Autodesk Inventor part; units mm, degrees
(part 2 of 2)
sketch "Sketch23" plane through (-20, 0, 0) normal (-1, 0, 0) x (0, 0, 1)
  circle A0 centre (8.0719, -81.9132) radius 5.7664 projected
  circle A1 centre (83.0719, -81.9132) radius 3.9821 projected
  circle A2 centre (2.2876, 58.0868) radius 3 projected
  circle A3 centre (83.0715, 100.0868) radius 3 projected
  circle A4 centre (83.0715, 260.0868) radius 3 projected
  circle A5 centre (8.0719, 243.0868) radius 2.5 projected
  circle A6 centre (37.6815, 343.0868) radius 3 projected
  circle A7 centre (83.0719, 348.0868) radius 6.7103 projected
  point P0 (0, 0)
extrude "Extrusion27" add sketch "Sketch23" against normal up to surface (20 mm away)
sketch "Sketch24" plane through (0, 0, 0) normal (1, 0, 0) x (0, 0, -1)
  arc A0 (-0.5719, 198.2351) -> (-0.5719, 217.9385) centre (-2.2876, 208.0868) ccw
  circle A1 centre (-2.2876, 208.0868) radius 10 projected
  point P0 (0, 0)
  constraints: 2 point on circle, 1 centre point, 4 other
ref_plane "Work Plane2" through (15, -91.9132, -7.7124) normal (-1, 0, 0) x (0, 0, 1)
extrude "Extrusion28" cut sketch "Sketch24" along normal up to surface (15 mm away)
sketch "Sketch25" plane through (-20, 0, 0) normal (-1, 0, 0) x (0, 0, 1)
  circle A0 centre (45.5719, -58.1139) radius 2.7
  circle A1 centre (45.5719, 80.6015) radius 2.6
  circle A2 centre (45.5719, 251.5868) radius 2.6
  circle A3 centre (45.5719, 251.5868) radius 5
  circle A4 centre (45.5719, 80.6015) radius 5
  circle A5 centre (45.5719, -58.1139) radius 5
  circle A6 centre (37.6815, 343.0868) radius 2.5
  circle A7 centre (83.0719, 348.0868) radius 2.5
  line L0 (26.8981, 333.0868) -> (64.2457, 333.0868)
  line L1 (47.3608, 292.8448) -> (66.0345, 330.1924)
  line L2 (25.1093, 330.1924) -> (43.783, 292.8448)
  line L3 (47.3608, 292.8448) -> (42.5596, 283.2426)
  line L4 (43.783, 292.8448) -> (48.6607, 283.0896)
  line L5 (45.5719, 333.0868) -> (45.5719, 289.2671)
  line L6 (45.5719, 251.5868) -> (55.5719, 251.5868)
  line L7 (45.5719, 251.5868) -> (35.5719, 251.5868)
  line L8 (55.5719, 80.6015) -> (35.5719, 80.6015)
  line L9 (45.5719, -58.1139) -> (55.5719, -58.1139)
  line L10 (55.5719, -58.1139) -> (35.5719, -58.1139)
  line L11 (35.5719, 251.5868) -> (55.5719, 251.5868) construction
  line L12 (35.5719, 256.5868) -> (55.5719, 256.5868)
  line L13 (55.5719, 246.5868) -> (35.5719, 246.5868)
  arc A8 (35.5719, 256.5868) -> (35.5719, 246.5868) centre (35.5719, 251.5868) ccw
  arc A9 (55.5719, 246.5868) -> (55.5719, 256.5868) centre (55.5719, 251.5868) ccw
  line L14 (35.5719, 80.6015) -> (55.5719, 80.6015) construction
  line L15 (35.5719, 85.6015) -> (55.5719, 85.6015)
  line L16 (55.5719, 75.6015) -> (35.5719, 75.6015)
  arc A10 (35.5719, 85.6015) -> (35.5719, 75.6015) centre (35.5719, 80.6015) ccw
  arc A11 (55.5719, 75.6015) -> (55.5719, 85.6015) centre (55.5719, 80.6015) ccw
  line L17 (35.5719, -58.1139) -> (55.5719, -58.1139) construction
  line L18 (35.5719, -53.1139) -> (55.5719, -53.1139)
  line L19 (55.5719, -63.1139) -> (35.5719, -63.1139)
  arc A12 (35.5719, -53.1139) -> (35.5719, -63.1139) centre (35.5719, -58.1139) ccw
  arc A13 (55.5719, -63.1139) -> (55.5719, -53.1139) centre (55.5719, -58.1139) ccw
  line L20 (35.5719, 251.5868) -> (55.5719, 251.5868) construction
  line L21 (35.5719, 254.1868) -> (55.5719, 254.1868)
  line L22 (55.5719, 248.9868) -> (35.5719, 248.9868)
  arc A14 (35.5719, 254.1868) -> (35.5719, 248.9868) centre (35.5719, 251.5868) ccw
  arc A15 (55.5719, 248.9868) -> (55.5719, 254.1868) centre (55.5719, 251.5868) ccw
  line L23 (55.5719, 80.6015) -> (35.5719, 80.6015) construction
  line L24 (55.5719, 83.2015) -> (35.5719, 83.2015)
  line L25 (35.5719, 78.0015) -> (55.5719, 78.0015)
  arc A16 (55.5719, 78.0015) -> (55.5719, 83.2015) centre (55.5719, 80.6015) ccw
  arc A17 (35.5719, 83.2015) -> (35.5719, 78.0015) centre (35.5719, 80.6015) ccw
  line L26 (35.5719, -58.1139) -> (55.5719, -58.1139) construction
  line L27 (35.5719, -55.4139) -> (55.5719, -55.4139)
  line L28 (55.5719, -60.8139) -> (35.5719, -60.8139)
  arc A18 (35.5719, -55.4139) -> (35.5719, -60.8139) centre (35.5719, -58.1139) ccw
  arc A19 (55.5719, -60.8139) -> (55.5719, -55.4139) centre (55.5719, -58.1139) ccw
  point P0 (0, 0)
  point P1 (45.5719, 80.6015)
  point P2 (45.5719, -58.1139)
  point P3 (45.5719, 80.6015)
  point P4 (45.5719, -58.1139)
  dimension "d126" = 10
  dimension "d127" = 10
  dimension "d128" = 10
  dimension "d129" = 10
  dimension "d130" = 10
  constraints: 70 end point, 24 point on circle, 24 tangent, 20 centre point, 7 collinear, 7 midpoint, 7 parallel, 5 horizontal, 3 coincident, 3 point on line, 18 other
  measures "d126" diameter of A3
  measures "d127" diameter of A4
  measures "d128" diameter of A5
  measures "d129" distance of L6.start L6.end
  measures "d130" distance of L6.start L7.end
extrude "Extrusion29" cut sketch "Sketch25" against normal through all contours L9 L10 A0 | L9 A5 L28 A0 | A0 L10 L9 | A0 L27 A5 L9 | A0 L10 A5 L27 | L28 A5 L10 A0 | A5 L27 A19 L28 | A5 L28 A18 L27 | L8 A1 | L8 A4 L25 A1 | A1 L24 A4 L8 | A1 L8 | A1 L8 A4 L24 | L25 A4 L8 A1 | A4 L24 A16 L25 | A4 L25 A17 L24 | L6 L7 A2 | L6 A3 L22 A2 | A2 L7 L6 | A2 L21 A3 L6 | A2 L7 A3 L21 | L22 A3 L7 A2 | A3 L21 A15 L22 | A3 L22 A14 L21
extrude "Extrusion30" cut sketch "Sketch25" against normal blind 11 contours L27 A5 | L28 A5 | L27 A18 L28 A5 L19 A12 L18 | A5 L18 A13 L19 L28 A19 L27 | L24 A4 | L25 A4 | A4 L15 A11 L16 L25 A16 L24 | L24 A17 L25 A4 L16 A10 L15 | L21 A3 | L22 A3 | L21 A14 L22 A3 L13 A8 L12 | A3 L12 A9 L13 L22 A15 L21
sketch "Sketch26" plane through (-20, 0, 0) normal (-1, 0, 0) x (0, 0, 1)
  line L0 (55.5719, -63.1139) -> (35.5719, -63.1139) projected
  arc A0 (35.5719, -53.1139) -> (35.5719, -63.1139) centre (35.5719, -58.1139) ccw projected
  line L1 (35.5719, -53.1139) -> (55.5719, -53.1139) projected
  arc A1 (55.5719, -63.1139) -> (55.5719, -53.1139) centre (55.5719, -58.1139) ccw projected
  line L2 (35.5719, 85.6015) -> (55.5719, 85.6015) projected
  arc A2 (55.5719, 75.6015) -> (55.5719, 85.6015) centre (55.5719, 80.6015) ccw projected
  line L3 (55.5719, 75.6015) -> (35.5719, 75.6015) projected
  arc A3 (35.5719, 85.6015) -> (35.5719, 75.6015) centre (35.5719, 80.6015) ccw projected
  line L4 (55.5719, 246.5868) -> (35.5719, 246.5868) projected
  arc A4 (35.5719, 256.5868) -> (35.5719, 246.5868) centre (35.5719, 251.5868) ccw projected
  line L5 (35.5719, 256.5868) -> (55.5719, 256.5868) projected
  arc A5 (55.5719, 246.5868) -> (55.5719, 256.5868) centre (55.5719, 251.5868) ccw projected
  circle A6 centre (2.2876, 208.0868) radius 3 projected
  circle A7 centre (37.6815, 23.0868) radius 3 projected
  circle A8 centre (37.6815, 183.0868) radius 3 projected
  line L6 (91.6177, -209.9132) -> (-3.4281, -209.9132) projected
  line L7 (118.5719, -179.5898) -> (91.6177, -209.9132) projected
  line L8 (118.5719, 480.8363) -> (118.5719, -179.5898) projected
  line L9 (84.6218, 518.7753) -> (118.5719, 480.8363) projected
  line L10 (-3.4281, 219.4525) -> (84.6218, 518.7753) projected
  line L11 (-3.4281, -209.9132) -> (-3.4281, 219.4525) projected
  point P0 (0, 0)
extrude "Extrusion31" add sketch "Sketch26" against normal up to surface (20 mm away) contours A6 | A7 | A8
sketch "Sketch27" plane through (15, 23.0868, 37.6815) normal (1, 0, 0) x (0, 0, -1)
  circle A0 centre (0, 0) radius 10 projected
  circle A1 centre (0, 160) radius 10 projected
  point P0 (37.6815, -23.0868)
extrude "Extrusion32" cut sketch "Sketch27" against normal up to surface (15 mm away)
sketch "Sketch28" plane through (0, -187.1938, 138.5719) normal (0, 0, 1) x (1, 0, 0)
  line L0 (75, 0) -> (75, 675.6721) projected
  line L1 (0, 675.6721) -> (75, 675.6721) projected
  line L2 (0, 0) -> (0, 675.6721) projected
  line L3 (0, 0) -> (75, 0) projected
  arc A0 (57, 649.6721) -> (57, 641.6721) centre (57, 645.6721) ccw projected
  line L4 (57, 649.6721) -> (67, 649.6721) projected
  arc A1 (67, 641.6721) -> (67, 649.6721) centre (67, 645.6721) ccw projected
  line L5 (67, 641.6721) -> (57, 641.6721) projected
  arc A2 (57, 672.1821) -> (57, 664.1821) centre (57, 668.1821) ccw projected
  line L6 (57, 672.1821) -> (67, 672.1821) projected
  arc A3 (67, 664.1821) -> (67, 672.1821) centre (67, 668.1821) ccw projected
  line L7 (67, 664.1821) -> (57, 664.1821) projected
  line L8 (75, 14.7186) -> (75, 14.7186) projected
  line L9 (75, 351.3416) -> (0, 351.3416)
  line L10 (0, 10.2186) -> (0, 665.4417) projected
  line L11 (67, 647.7721) -> (57, 647.7721) projected
  arc A4 (57, 647.7721) -> (57, 643.5721) centre (57, 645.6721) ccw projected
  line L12 (57, 643.5721) -> (67, 643.5721) projected
  arc A5 (67, 643.5721) -> (67, 647.7721) centre (67, 645.6721) ccw projected
  line L13 (53, 645.6721) -> (53, 351.3416)
  arc A6 (67, 641.6721) -> (67, 649.6721) centre (67, 645.6721) ccw projected
  line L14 (71, 645.6721) -> (71, 351.3416)
  line L15 (71, 355.6306) -> (53, 355.6306) construction
  line L16 (67, 359.6306) -> (57, 359.6306)
  line L17 (57, 351.6306) -> (67, 351.6306)
  arc A7 (67, 351.6306) -> (67, 359.6306) centre (67, 355.6306) ccw
  arc A8 (57, 359.6306) -> (57, 351.6306) centre (57, 355.6306) ccw
  line L18 (67, 645.6721) -> (67, 340.473)
  arc A9 (57, 647.7721) -> (57, 643.5721) centre (57, 645.6721) ccw projected
  line L19 (57, 645.6721) -> (57, 335.2008)
  line L20 (67, 355.6306) -> (57, 355.6306) construction
  line L21 (67, 357.7306) -> (57, 357.7306)
  line L22 (57, 353.5306) -> (67, 353.5306)
  arc A10 (67, 353.5306) -> (67, 357.7306) centre (67, 355.6306) ccw
  arc A11 (57, 357.7306) -> (57, 353.5306) centre (57, 355.6306) ccw
  line L23 (71, 498.5068) -> (53, 498.5068) construction
  line L24 (67, 502.5068) -> (57, 502.5068)
  line L25 (57, 494.5068) -> (67, 494.5068)
  arc A12 (67, 494.5068) -> (67, 502.5068) centre (67, 498.5068) ccw
  arc A13 (57, 502.5068) -> (57, 494.5068) centre (57, 498.5068) ccw
  line L26 (67, 498.5068) -> (57, 498.5068) construction
  line L27 (67, 500.6068) -> (57, 500.6068)
  line L28 (57, 496.4068) -> (67, 496.4068)
  arc A14 (67, 496.4068) -> (67, 500.6068) centre (67, 498.5068) ccw
  arc A15 (57, 500.6068) -> (57, 496.4068) centre (57, 498.5068) ccw
  line L29 (71, 351.3416) -> (71, 0)
  line L30 (67, 340.473) -> (67, 0)
  line L31 (57, 335.2008) -> (57, 0)
  line L32 (0, 0) -> (75, 0) projected
  line L33 (53, 351.3416) -> (53, 0)
  line L34 (71, 10.2186) -> (53, 10.2186) construction
  line L35 (67, 14.2186) -> (57, 14.2186)
  line L36 (57, 6.2186) -> (67, 6.2186)
  arc A16 (67, 6.2186) -> (67, 14.2186) centre (67, 10.2186) ccw
  arc A17 (57, 14.2186) -> (57, 6.2186) centre (57, 10.2186) ccw
  line L37 (67, 10.2186) -> (57, 10.2186) construction
  line L38 (67, 12.3186) -> (57, 12.3186)
  line L39 (57, 8.1186) -> (67, 8.1186)
  arc A18 (67, 8.1186) -> (67, 12.3186) centre (67, 10.2186) ccw
  arc A19 (57, 12.3186) -> (57, 8.1186) centre (57, 10.2186) ccw
  line L40 (67, 117.3266) -> (57, 117.3266) construction
  line L41 (67, 119.4266) -> (57, 119.4266)
  line L42 (57, 115.2266) -> (67, 115.2266)
  arc A20 (67, 115.2266) -> (67, 119.4266) centre (67, 117.3266) ccw
  arc A21 (57, 119.4266) -> (57, 115.2266) centre (57, 117.3266) ccw
  line L43 (71, 117.3266) -> (53, 117.3266) construction
  line L44 (67, 121.3266) -> (57, 121.3266)
  line L45 (57, 113.3266) -> (67, 113.3266)
  arc A22 (67, 113.3266) -> (67, 121.3266) centre (67, 117.3266) ccw
  arc A23 (57, 121.3266) -> (57, 113.3266) centre (57, 117.3266) ccw
  line L46 (62, 121.3266) -> (62, 351.6306)
  line L47 (71, 236.4786) -> (53, 236.4786) construction
  line L48 (67, 240.4786) -> (57, 240.4786)
  line L49 (57, 232.4786) -> (67, 232.4786)
  arc A24 (67, 232.4786) -> (67, 240.4786) centre (67, 236.4786) ccw
  arc A25 (57, 240.4786) -> (57, 232.4786) centre (57, 236.4786) ccw
  line L50 (67, 236.4786) -> (57, 236.4786) construction
  line L51 (67, 238.5786) -> (57, 238.5786)
  line L52 (57, 234.3786) -> (67, 234.3786)
  arc A26 (67, 234.3786) -> (67, 238.5786) centre (67, 236.4786) ccw
  arc A27 (57, 238.5786) -> (57, 234.3786) centre (57, 236.4786) ccw
  point P0 (0, 187.1938)
  point P1 (37.5, 675.6721)
  point P2 (37.5, 0)
  point P3 (75, 687.9645)
  point P4 (62, 355.6306)
  point P5 (62, 355.6306)
  point P6 (62, 498.5068)
  point P7 (62, 498.5068)
  point P8 (62, 10.2186)
  point P9 (62, 10.2186)
  point P10 (62, 117.3266)
  point P11 (62, 117.3266)
  point P12 (62, 236.4786)
  point P13 (62, 236.4786)
  dimension "d139" = 675.6721
  dimension "d140" = 8
  dimension "d141" = 4.2
  dimension "d142" = 8
  dimension "d143" = 4.2
  dimension "d144" = 8
  dimension "d145" = 4.2
  dimension "d146" = 4.2
  dimension "d147" = 8
  dimension "d148" = 8
  dimension "d149" = 4.2
  constraints: 100 end point, 53 point on circle, 41 tangent, 27 point on line, 20 centre point, 16 midpoint, 13 perpendicular, 12 parallel, 3 collinear, 2 other
  measures "d139" distance of point (37.5, 675.672) point (37.5, 0)
  measures "d140" diameter of A8
  measures "d141" diameter of A11
  measures "d142" diameter of A13
  measures "d143" diameter of A15
  measures "d144" diameter of A17
  measures "d145" diameter of A19
  measures "d146" diameter of A21
  measures "d147" diameter of A23
  measures "d148" diameter of A25
  measures "d149" diameter of A27
extrude "Extrusion33" cut sketch "Sketch28" against normal through all contours L39 L31 L38 L30 | L30 A18 | L22 L19 L21 L18 | L18 A10 | L52 L46 L51 L30 | L30 A26 | A19 L31 | L42 L31 L41 L30 | L30 A20 | L46 L52 L31 L51 | A11 L19 | L28 L19 L27 L18 | L18 A14 | A21 L31 | L31 A27 | A15 L19
extrude "Extrusion34" cut sketch "Sketch28" against normal up to surface (8 mm away) contours A16 L30 A18 | A7 L18 A10 | A24 L30 A26 | L36 L31 L39 L30 | A22 L30 A20 | L30 L38 L31 L35 | L17 L19 L22 L18 | A12 L18 A14 | L18 L21 L19 L16 | L49 L46 L52 L30 | L30 L51 L46 L48 | A17 L31 A19 | L39 L31 L38 L30 | L30 A18 | L45 L31 L42 L30 | L30 L41 L31 L44 | L46 L51 L31 L48 | L22 L19 L21 L18 | L18 A10 | L25 L19 L28 L18 | L18 L27 L19 L24 | L19 A11 A8 | L52 L46 L51 L30 | L30 A26 | L49 L31 L52 L46 | A19 L31 | L42 L31 L41 L30 | L30 A20 | A23 L31 A21 | L46 L52 L31 L51 | L31 A27 A25 | A11 L19 | L28 L19 L27 L18 | L18 A14 | A13 L19 A15 | A21 L31 | L31 A27 | A15 L19
sketch "Sketch29" plane through (75, 498.5358, 127.5719) normal (0, 0, -1) x (-1, 0, 0)
  arc A0 (8, -447.151) -> (8, -451.351) centre (8, -449.251) ccw projected
  line L0 (8, -447.151) -> (18, -447.151) projected
  arc A1 (18, -451.351) -> (18, -447.151) centre (18, -449.251) ccw projected
  line L1 (18, -451.351) -> (8, -451.351) projected
  line L2 (8, -566.303) -> (18, -566.303) projected
  arc A2 (18, -570.503) -> (18, -566.303) centre (18, -568.403) ccw projected
  line L3 (18, -570.503) -> (8, -570.503) projected
  arc A3 (8, -566.303) -> (8, -570.503) centre (8, -568.403) ccw projected
  arc A4 (18, -332.199) -> (18, -327.999) centre (18, -330.099) ccw projected
  line L4 (18, -332.199) -> (8, -332.199) projected
  arc A5 (8, -327.999) -> (8, -332.199) centre (8, -330.099) ccw projected
  line L5 (8, -327.999) -> (18, -327.999) projected
  arc A6 (18, -189.3227) -> (18, -185.1227) centre (18, -187.2227) ccw projected
  line L6 (18, -189.3227) -> (8, -189.3227) projected
  arc A7 (8, -185.1227) -> (8, -189.3227) centre (8, -187.2227) ccw projected
  line L7 (8, -185.1227) -> (18, -185.1227) projected
  line L8 (18, -19.6474) -> (8, -19.6474) projected
  arc A8 (8, -15.4474) -> (8, -19.6474) centre (8, -17.5474) ccw projected
  line L9 (8, -15.4474) -> (18, -15.4474) projected
  arc A9 (18, -19.6474) -> (18, -15.4474) centre (18, -17.5474) ccw projected
  line L10 (18, -42.1575) -> (8, -42.1575) projected
  arc A10 (8, -37.9575) -> (8, -42.1575) centre (8, -40.0575) ccw projected
  line L11 (8, -37.9575) -> (18, -37.9575) projected
  arc A11 (18, -42.1575) -> (18, -37.9575) centre (18, -40.0575) ccw projected
  line L12 (28, -671.0109) -> (0, -671.0109) projected
  line L13 (28, 2.235) -> (28, -671.0109) projected
  line L14 (28, 2.235) -> (0, 2.235) projected
  line L15 (0, -671.0109) -> (0, 2.235) projected
  line L16 (28, -671.0109) -> (0, -671.0109) projected
  line L17 (0, -685.7295) -> (0, -10.0575) projected
  line L18 (28, -671.0109) -> (0, -671.0109)
  line L19 (0, -671.0109) -> (0, -685.7295)
  line L20 (0, -685.7295) -> (28, -685.7295)
  line L21 (28, -685.7295) -> (28, -671.0109)
  line L22 (0, -710.449) -> (0, -671.0109) projected
  line L23 (28, -671.0109) -> (0, -671.0109)
  line L24 (0, -671.0109) -> (0, -682.3863)
  line L25 (0, -682.3863) -> (28, -682.3863)
  line L26 (28, -682.3863) -> (28, -671.0109)
  point P0 (75, -498.5358)
  constraints: 16 end point, 4 parallel, 2 horizontal, 2 perpendicular, 1 point on line
extrude "Extrusion35" cut sketch "Sketch29" along normal through all contours L21 L25 L17 L12
sketch "Sketch30" plane through (0, 0, 0) normal (1, 0, 0) x (0, 0, -1)
  circle A0 centre (-45.5719, -58.1139) radius 2.7
  circle A1 centre (-83.0719, -81.9132) radius 2.5
  circle A2 centre (-8.0719, -81.9132) radius 2.5
  circle A3 centre (-45.5719, 80.6015) radius 2.6
  circle A4 centre (-83.0715, 100.0868) radius 2.5
  circle A5 centre (-2.2876, 58.0868) radius 2.5
  circle A6 centre (-8.0719, 243.0868) radius 2.5
  circle A7 centre (-45.5719, 251.5868) radius 2.0092
  circle A8 centre (-83.0715, 260.0868) radius 2.5
  line L0 (-117.4605, -183.8505) -> (-127.5719, -183.8505) projected
  line L1 (-127.5719, -183.8505) -> (-127.5719, 500.7708) projected
  line L2 (-127.5719, 500.7708) -> (-138.5719, 488.4783) projected
  line L3 (-138.5719, -187.1938) -> (-138.5719, 488.4783) projected
  line L4 (-100.599, -229.9132) -> (-138.5719, -187.1938) projected
  line L5 (23.4281, -229.9132) -> (-100.599, -229.9132) projected
  line L6 (23.4281, -211.9132) -> (23.4281, -229.9132) projected
  line L7 (-92.5159, -211.9132) -> (23.4281, -211.9132) projected
  line L8 (-92.5159, -211.9132) -> (-117.4605, -183.8505) projected
  line L9 (-35.5719, -60.8139) -> (-55.5719, -60.8139) projected
  arc A9 (-55.5719, -55.4139) -> (-55.5719, -60.8139) centre (-55.5719, -58.1139) ccw projected
  line L10 (-55.5719, -55.4139) -> (-35.5719, -55.4139) projected
  arc A10 (-35.5719, -60.8139) -> (-35.5719, -55.4139) centre (-35.5719, -58.1139) ccw projected
  line L11 (-55.5719, 83.2015) -> (-35.5719, 83.2015) projected
  arc A11 (-35.5719, 78.0015) -> (-35.5719, 83.2015) centre (-35.5719, 80.6015) ccw projected
  line L12 (-35.5719, 78.0015) -> (-55.5719, 78.0015) projected
  arc A12 (-55.5719, 83.2015) -> (-55.5719, 78.0015) centre (-55.5719, 80.6015) ccw projected
  line L13 (-35.5719, 248.9868) -> (-55.5719, 248.9868) projected
  arc A13 (-55.5719, 254.1868) -> (-55.5719, 248.9868) centre (-55.5719, 251.5868) ccw projected
  line L14 (-55.5719, 254.1868) -> (-35.5719, 254.1868) projected
  arc A14 (-35.5719, 248.9868) -> (-35.5719, 254.1868) centre (-35.5719, 251.5868) ccw projected
  line L15 (-123.5719, -176.9752) -> (-123.5719, 478.248) projected
  line L16 (-92.5159, -211.9132) -> (-123.5719, -176.9752) projected
  line L17 (23.4281, -211.9132) -> (-92.5159, -211.9132) projected
  line L18 (23.4281, -211.9132) -> (23.4281, 222.3331) projected
  line L19 (23.4281, 222.3331) -> (-75.5719, 558.8805) projected
  line L20 (-76.4445, 557.9054) -> (-75.5719, 558.8805) projected
  arc A15 (-75.5719, 557.572) -> (-76.4445, 557.9054) centre (-76.0719, 557.572) ccw projected
  line L21 (-75.5719, 554.0258) -> (-75.5719, 557.572) projected
  arc A16 (-75.6497, 553.7579) -> (-75.5719, 554.0258) centre (-76.0719, 554.0258) ccw projected
  line L22 (-123.5719, 478.248) -> (-75.6497, 553.7579) projected
  line L23 (-110.2837, 493.0975) -> (-110.2933, 493.0868) projected
  line L24 (-110.2837, 493.0975) -> (-110.2717, 493.0868) projected
  line L25 (-110.2717, 493.0868) -> (-110.2933, 493.0868) projected
  line L26 (-127.5719, -47.274) -> (-16.9685, -0.267)
  line L27 (-123.5719, 478.248) -> (-123.5719, -176.9752) projected
  line L28 (-123.5719, -45.574) -> (-166.4144, -45.574)
  line L29 (-123.5719, 128.4564) -> (-162.2034, 128.4564)
  line L30 (-166.4144, 328.3013) -> (-123.5719, 328.3013)
  line L31 (-118.5719, 480.8363) -> (-118.5719, -179.5898) projected
  line L32 (23.4281, -229.9132) -> (-100.599, -229.9132) projected
  line L33 (23.4281, -229.9132) -> (-16.5719, -229.9132)
  line L34 (23.4281, 222.3331) -> (-75.5719, 558.8805) projected
  line L35 (-16.9685, -0.267) -> (51.1207, -0.267)
  line L36 (-16.9685, 166.07) -> (46.6618, 166.07)
  line L37 (-16.9685, 166.07) -> (-127.5719, 127.045)
  line L38 (-89.4582, 338.3363) -> (-49.4582, 338.3363)
  line L39 (-49.4582, 338.3363) -> (-49.4582, 350.1029)
  line L40 (-5.5719, 363.0126) -> (-49.4582, 350.1029)
  line L41 (-89.4582, 338.3363) -> (-123.5719, 328.3013)
  line L42 (35.4331, -0.267) -> (41.6219, -293.9707)
  line L43 (41.6219, -293.9707) -> (-179.8832, -298.6381)
  line L44 (-179.8832, -298.6381) -> (-166.4144, -45.574)
  line L45 (-166.4144, -45.574) -> (-162.2034, 128.4564)
  line L46 (46.6618, 166.07) -> (35.4331, -0.267)
  line L47 (46.6618, 166.07) -> (43.1382, 333.2916)
  line L48 (43.1382, 333.2916) -> (-5.5719, 363.0126)
  line L49 (-166.4144, 328.3013) -> (-162.2034, 128.4564)
  line L50 (-5.5719, 363.0126) -> (-64.3515, 609.6406)
  line L51 (-64.3515, 609.6406) -> (-157.0112, 504.9789)
  line L52 (-157.0112, 504.9789) -> (-166.4144, 328.3013)
  point P0 (0, 0)
  point P1 (23.4281, -0.267)
  point P2 (-16.9685, 359.6602)
  dimension "d156" = 40
  dimension "d157" = 40
  constraints: 46 end point, 9 centre point, 9 point on line, 5 perpendicular, 3 horizontal, 2 parallel, 18 other
  measures "d156" distance of L5.start L33.end
  measures "d157" distance of L38.start L38.end
extrude "Extrusion36" cut sketch "Sketch30" along normal through all both and the other way through all contours A1 | A2 | A4 | A5 | A6 | A8 | L8 L7 L6 L5 L4 L3 L28 L1 L0 | L16 L15 L26 L35 L18 L7 L8 | L0 L1 L26 L15 L16 | L1 L28 L26 | L18 L35 L42 L43 L44 L28 L3 L4 L5 L6 | L28 L1 L37 L15 | L15 L37 L31 L26 | L28 L3 L29 L1 | L35 L26 L31 L37 L36 L18 | L29 L1 L30 L15 | L37 L1 L29 | L15 L41 L31 L37 | L28 L45 L29 L3 | L36 L37 L31 L41 L38 L39 L40 L19 L18 | L29 L3 L30 L1 | L29 L49 L30 L3
sketch "Sketch31" plane through (0, 328.3013, 138.5719) normal (0, -1, 0) x (1, 0, 0)
  circle A0 centre (39.8089, -7.5) radius 5.25 projected
  circle A1 centre (5.2738, -7.5) radius 3.5 projected
  arc A2 (67.5, -8) -> (67.5, -3) centre (67.5, -5.5) ccw projected
  line L0 (67.5, -3) -> (52.5, -3) projected
  arc A3 (52.5, -3) -> (52.5, -8) centre (52.5, -5.5) ccw projected
  line L1 (52.5, -8) -> (67.5, -8) projected
  line L2 (0, 0) -> (-15, -15) projected
  line L3 (75, 0) -> (0, 0) projected
  line L4 (75, -11) -> (75, 0) projected
  line L5 (47, -11) -> (75, -11) projected
  line L6 (47, -15) -> (47, -11) projected
  line L7 (0, -15) -> (47, -15) projected
  line L8 (-15, -15) -> (0, -15) projected
  circle A4 centre (20.6486, -7.5) radius 5.25 projected
  line L9 (52.5, -5.5) -> (67.5, -5.5) construction
  line L10 (52.5, -8.75) -> (67.5, -8.75)
  line L11 (67.5, -2.25) -> (52.5, -2.25)
  arc A5 (52.5, -2.25) -> (52.5, -8.75) centre (52.5, -5.5) ccw
  arc A6 (67.5, -8.75) -> (67.5, -2.25) centre (67.5, -5.5) ccw
  circle A7 centre (39.8089, -7.5) radius 3.5
  circle A8 centre (20.6486, -7.5) radius 3.5
  circle A9 centre (5.2738, -7.5) radius 4.25
  point P0 (0, -138.5719)
  point P1 (60, -5.5)
  dimension "d160" = 6.5
  dimension "d161" = 7
  dimension "d162" = 7
  dimension "d163" = 8.5
  constraints: 8 end point, 5 centre point, 4 point on circle, 4 tangent, 3 coincident, 1 horizontal, 1 midpoint, 1 parallel
  measures "d160" diameter of A6
  measures "d161" diameter of A7
  measures "d162" diameter of A8
  measures "d163" diameter of A9
extrude "Extrusion37" cut sketch "Sketch31" against normal blind 15 contours A1 | L1 A3 L0 A2 | A5 L11 A6 L10 | A9
sketch "Sketch32" plane through (0, 328.3013, 138.5719) normal (0, -1, 0) x (1, 0, 0)
  circle A0 centre (39.8089, -7.5) radius 5.25 projected
  circle A1 centre (5.2738, -7.5) radius 3.5 projected
  arc A2 (67.5, -8) -> (67.5, -3) centre (67.5, -5.5) ccw projected
  line L0 (67.5, -3) -> (52.5, -3) projected
  arc A3 (52.5, -3) -> (52.5, -8) centre (52.5, -5.5) ccw projected
  line L1 (52.5, -8) -> (67.5, -8) projected
  line L2 (0, 0) -> (-15, -15) projected
  line L3 (75, 0) -> (0, 0) projected
  line L4 (75, -11) -> (75, 0) projected
  line L5 (47, -11) -> (75, -11) projected
  line L6 (47, -15) -> (47, -11) projected
  line L7 (0, -15) -> (47, -15) projected
  line L8 (-15, -15) -> (0, -15) projected
  circle A4 centre (20.6486, -7.5) radius 5.25 projected
  circle A5 centre (20.6486, -7.5) radius 3.5
  circle A6 centre (39.8089, -7.5) radius 3.5
  point P0 (0, -138.5719)
  dimension "d166" = 7
  dimension "d167" = 7
  constraints: 2 centre point, 2 coincident
  measures "d166" diameter of A5
  measures "d167" diameter of A6
extrude "Extrusion38" add sketch "Sketch32" along normal blind 10 contours A5 | A6
chamfer "Chamfer4" distance 1 angle 45 7 edges at (60, 328.3013, 129.8219) (49.25, 328.3013, 133.0719) (60, 328.3013, 136.3219) (70.75, 328.3013, 133.0719) (36.3089, 318.3013, 131.0719) (17.1486, 318.3013, 131.0719) (1.0238, 328.3013, 131.0719)
sketch "Sketch33" plane through (0, 338.3363, 49.4582) normal (0, -1, 0) x (1, 0, 0)
  line L0 (-15, 30.3447) -> (-15, 9.6553) projected
  arc A0 (-15, 9.6553) -> (-5, 9.6553) centre (-10, 9.6553) ccw projected
  line L1 (-5, 9.6553) -> (-5, 30.3447) projected
  arc A1 (-5, 30.3447) -> (-15, 30.3447) centre (-10, 30.3447) ccw projected
  line L2 (-20, 40) -> (-20, 0) projected
  line L3 (0, 40) -> (-20, 40) projected
  line L4 (0, 0) -> (0, 40) projected
  line L5 (-20, 0) -> (0, 0) projected
  line L6 (-10, 9.6553) -> (-10, 30.3447) construction
  line L7 (-4.25, 9.6553) -> (-4.25, 30.3447)
  line L8 (-15.75, 30.3447) -> (-15.75, 9.6553)
  arc A2 (-15.75, 9.6553) -> (-4.25, 9.6553) centre (-10, 9.6553) ccw
  arc A3 (-4.25, 30.3447) -> (-15.75, 30.3447) centre (-10, 30.3447) ccw
  point P0 (0, -49.4582)
  point P1 (-10, 20)
  dimension "d173" = 11.5
  constraints: 8 end point, 4 point on circle, 4 tangent, 2 centre point, 1 midpoint, 1 parallel, 1 vertical
  measures "d173" diameter of A3
extrude "Extrusion39" cut sketch "Sketch33" against normal blind 15 contours A1 L1 A0 L0 | A2 L8 A3 L7
chamfer "Chamfer5" distance 1 angle 45 4 edges at (-4.25, 338.3363, 69.4582) (-10, 338.3363, 53.3635) (-15.75, 338.3363, 69.4582) (-10, 338.3363, 85.5529)
body "Solid1"
